Autodesk Inventor part; units mm, degrees
(part 2 of 2)
  line L549 (-543.4229, 5.588) -> (-545.3351, 0.3343)
  arc A272 (-545.8125, 0) -> (-545.3351, 0.3343) centre (-545.8125, 0.508) ccw
  line L550 (-545.8125, 0) -> (-547.3989, 0)
  arc A273 (-547.8763, 0.3343) -> (-547.3989, 0) centre (-547.3989, 0.508) ccw
  line L551 (-547.8763, 0.3343) -> (-549.7885, 5.588)
  arc A274 (-539.8966, 0.3343) -> (-539.4193, 0) centre (-539.4193, 0.508) ccw
  line L552 (-537.8328, 0) -> (-539.4193, 0)
  arc A275 (-537.8328, 0) -> (-537.3555, 0.3343) centre (-537.8328, 0.508) ccw
  line L553 (-535.4433, 5.588) -> (-537.3555, 0.3343)
  line L554 (-543.4229, 5.588) -> (-541.8088, 5.588)
  line L555 (-547.8763, 0.3343) -> (-549.7885, 5.588)
  line L556 (-554.5854, 0) -> (-546.6057, 0) construction
  line L557 (-551.4026, 5.588) -> (-553.3148, 0.3343)
  arc A276 (-553.7921, 0) -> (-553.3148, 0.3343) centre (-553.7921, 0.508) ccw
  line L558 (-553.7921, 0) -> (-555.3786, 0)
  arc A277 (-555.8559, 0.3343) -> (-555.3786, 0) centre (-555.3786, 0.508) ccw
  line L559 (-555.8559, 0.3343) -> (-557.7681, 5.588)
  arc A278 (-547.8763, 0.3343) -> (-547.3989, 0) centre (-547.3989, 0.508) ccw
  line L560 (-545.8125, 0) -> (-547.3989, 0)
  arc A279 (-545.8125, 0) -> (-545.3351, 0.3343) centre (-545.8125, 0.508) ccw
  line L561 (-543.4229, 5.588) -> (-545.3351, 0.3343)
  line L562 (-551.4026, 5.588) -> (-549.7885, 5.588)
  line L563 (7.1726, 38.1) -> (7.1726, 44.1)
  line L564 (7.1726, 44.1) -> (19.8726, 44.1)
  line L565 (19.8726, 44.1) -> (19.8726, -6)
  line L566 (19.8726, -6) -> (7.1726, -6)
  line L567 (7.1726, -6) -> (7.1726, 0)
  line L568 (4.783, 0) -> (7.1726, 0)
  point P0 (0, 0)
  point P1 (0, 0)
  point P2 (0, 5.588)
  point P3 (0, 0)
  point P4 (-7.9796, 5.588)
  point P5 (-7.9796, 0)
  point P6 (-7.9796, 0)
  point P7 (-7.9796, 0)
  point P8 (-15.9593, 5.588)
  point P9 (-15.9593, 0)
  point P10 (-15.9593, 0)
  point P11 (-15.9593, 0)
  point P12 (-23.9389, 5.588)
  point P13 (-23.9389, 0)
  point P14 (-23.9389, 0)
  point P15 (-23.9389, 0)
  point P16 (-31.9186, 5.588)
  point P17 (-31.9186, 0)
  point P18 (-31.9186, 0)
  point P19 (-31.9186, 0)
  point P20 (-39.8982, 5.588)
  point P21 (-39.8982, 0)
  point P22 (-39.8982, 0)
  point P23 (-39.8982, 0)
  point P24 (-47.8779, 5.588)
  point P25 (-47.8779, 0)
  point P26 (-47.8779, 0)
  point P27 (-47.8779, 0)
  point P28 (-55.8575, 5.588)
  point P29 (-55.8575, 0)
  point P30 (-55.8575, 0)
  point P31 (-55.8575, 0)
  point P32 (-63.8372, 5.588)
  point P33 (-63.8372, 0)
  point P34 (-63.8372, 0)
  point P35 (-63.8372, 0)
  point P36 (-71.8168, 5.588)
  point P37 (-71.8168, 0)
  point P38 (-71.8168, 0)
  point P39 (-71.8168, 0)
  point P40 (-79.7965, 5.588)
  point P41 (-79.7965, 0)
  point P42 (-79.7965, 0)
  point P43 (-79.7965, 0)
  point P44 (-87.7761, 5.588)
  point P45 (-87.7761, 0)
  point P46 (-87.7761, 0)
  point P47 (-87.7761, 0)
  point P48 (-95.7557, 5.588)
  point P49 (-95.7557, 0)
  point P50 (-95.7557, 0)
  point P51 (-95.7557, 0)
  point P52 (-103.7354, 5.588)
  point P53 (-103.7354, 0)
  point P54 (-103.7354, 0)
  point P55 (-103.7354, 0)
  point P56 (-111.715, 5.588)
  point P57 (-111.715, 0)
  point P58 (-111.715, 0)
  point P59 (-111.715, 0)
  point P60 (-119.6947, 5.588)
  point P61 (-119.6947, 0)
  point P62 (-119.6947, 0)
  point P63 (-119.6947, 0)
  point P64 (-127.6743, 5.588)
  point P65 (-127.6743, 0)
  point P66 (-127.6743, 0)
  point P67 (-127.6743, 0)
  point P68 (-135.654, 5.588)
  point P69 (-135.654, 0)
  point P70 (-135.654, 0)
  point P71 (-135.654, 0)
  point P72 (-143.6336, 5.588)
  point P73 (-143.6336, 0)
  point P74 (-143.6336, 0)
  point P75 (-143.6336, 0)
  point P76 (-151.6133, 5.588)
  point P77 (-151.6133, 0)
  point P78 (-151.6133, 0)
  point P79 (-151.6133, 0)
  point P80 (-159.5929, 5.588)
  point P81 (-159.5929, 0)
  point P82 (-159.5929, 0)
  point P83 (-159.5929, 0)
  point P84 (-167.5726, 5.588)
  point P85 (-167.5726, 0)
  point P86 (-167.5726, 0)
  point P87 (-167.5726, 0)
  point P88 (-175.5522, 5.588)
  point P89 (-175.5522, 0)
  point P90 (-175.5522, 0)
  point P91 (-175.5522, 0)
  point P92 (-183.5318, 5.588)
  point P93 (-183.5318, 0)
  point P94 (-183.5318, 0)
  point P95 (-183.5318, 0)
  point P96 (-191.5115, 5.588)
  point P97 (-191.5115, 0)
  point P98 (-191.5115, 0)
  point P99 (-191.5115, 0)
  point P100 (-199.4911, 5.588)
  point P101 (-199.4911, 0)
  point P102 (-199.4911, 0)
  point P103 (-199.4911, 0)
  point P104 (-207.4708, 5.588)
  point P105 (-207.4708, 0)
  point P106 (-207.4708, 0)
  point P107 (-207.4708, 0)
  point P108 (-215.4504, 5.588)
  point P109 (-215.4504, 0)
  point P110 (-215.4504, 0)
  point P111 (-215.4504, 0)
  point P112 (-223.4301, 5.588)
  point P113 (-223.4301, 0)
  point P114 (-223.4301, 0)
  point P115 (-223.4301, 0)
  point P116 (-231.4097, 5.588)
  point P117 (-231.4097, 0)
  point P118 (-231.4097, 0)
  point P119 (-231.4097, 0)
  point P120 (-239.3894, 5.588)
  point P121 (-239.3894, 0)
  point P122 (-239.3894, 0)
  point P123 (-239.3894, 0)
  point P124 (-247.369, 5.588)
  point P125 (-247.369, 0)
  point P126 (-247.369, 0)
  point P127 (-247.369, 0)
  point P128 (-255.3487, 5.588)
  point P129 (-255.3487, 0)
  point P130 (-255.3487, 0)
  point P131 (-255.3487, 0)
  point P132 (-263.3283, 5.588)
  point P133 (-263.3283, 0)
  point P134 (-263.3283, 0)
  point P135 (-263.3283, 0)
  point P136 (-271.3079, 5.588)
  point P137 (-271.3079, 0)
  point P138 (-271.3079, 0)
  point P139 (-271.3079, 0)
  point P140 (-279.2876, 5.588)
  point P141 (-279.2876, 0)
  point P142 (-279.2876, 0)
  point P143 (-279.2876, 0)
  point P144 (-287.2672, 5.588)
  point P145 (-287.2672, 0)
  point P146 (-287.2672, 0)
  point P147 (-287.2672, 0)
  point P148 (-295.2469, 5.588)
  point P149 (-295.2469, 0)
  point P150 (-295.2469, 0)
  point P151 (-295.2469, 0)
  point P152 (-303.2265, 5.588)
  point P153 (-303.2265, 0)
  point P154 (-303.2265, 0)
  point P155 (-303.2265, 0)
  point P156 (-311.2062, 5.588)
  point P157 (-311.2062, 0)
  point P158 (-311.2062, 0)
  point P159 (-311.2062, 0)
  point P160 (-319.1858, 5.588)
  point P161 (-319.1858, 0)
  point P162 (-319.1858, 0)
  point P163 (-319.1858, 0)
  point P164 (-327.1655, 5.588)
  point P165 (-327.1655, 0)
  point P166 (-327.1655, 0)
  point P167 (-327.1655, 0)
  point P168 (-335.1451, 5.588)
  point P169 (-335.1451, 0)
  point P170 (-335.1451, 0)
  point P171 (-335.1451, 0)
  point P172 (-343.1247, 5.588)
  point P173 (-343.1247, 0)
  point P174 (-343.1247, 0)
  point P175 (-343.1247, 0)
  point P176 (-351.1044, 5.588)
  point P177 (-351.1044, 0)
  point P178 (-351.1044, 0)
  point P179 (-351.1044, 0)
  point P180 (-359.084, 5.588)
  point P181 (-359.084, 0)
  point P182 (-359.084, 0)
  point P183 (-359.084, 0)
  point P184 (-367.0637, 5.588)
  point P185 (-367.0637, 0)
  point P186 (-367.0637, 0)
  point P187 (-367.0637, 0)
  point P188 (-375.0433, 5.588)
  point P189 (-375.0433, 0)
  point P190 (-375.0433, 0)
  point P191 (-375.0433, 0)
  point P192 (-383.023, 5.588)
  point P193 (-383.023, 0)
  point P194 (-383.023, 0)
  point P195 (-383.023, 0)
  point P196 (-391.0026, 5.588)
  point P197 (-391.0026, 0)
  point P198 (-391.0026, 0)
  point P199 (-391.0026, 0)
  dimension "d15" = 40
  dimension "d16" = 40
  dimension "d17" = 40
  dimension "d18" = 5.588
  dimension "d19" = 0.508
  dimension "d20" = 7.9796
  dimension "d21" = 3.9898
  dimension "d22" = 1.6141
  dimension "d23" = 1.5864
  dimension "d27" = 7.9796
  dimension "d32" = 38.1
  dimension "d35" = 6
  dimension "d36" = 6
  dimension "d37" = 12.7
  constraints: 1138 end point, 560 point on circle, 280 centre point, 141 coincident, 8 tangent, 7 perpendicular, 4 horizontal alignment, 4 midpoint, 3 equal radius, 2 horizontal, 2 point on line, 2 vertical, 1 collinear, 1 vertical alignment, 2346 other
  measures "d15" angle of L4 L6
  measures "d16" angle of L2 L4
  measures "d17" angle of L0 L2
  measures "d18" distance between parallel lines of L1 L3
  measures "d19" radius of A3
  measures "d20" distance of L7.end L7.start
  measures "d21" horizontal distance of point (0, 5.588) L7.start
  measures "d22" distance of L4.start L2.end
  measures "d23" distance of A2.centre A3.centre
  measures "d27" distance of L2.end L11.end
  measures "d32" distance between parallel lines of L444 L9
  measures "d35" distance of L8.end L563.end
  measures "d36" distance from line of L1.start L566
  measures "d37" distance of L563.end L564.end
extrude "Extrusion1" add sketch "Sketch1" along normal blind 4.7625
sketch "Sketch2" plane through (0, 0, 4.7625) normal (0, 0, 1) x (1, 0, 0)
  line L0 (7.1726, 2.54) -> (-557.7681, 2.54) construction
  line L1 (-555.3786, 0) -> (-553.7921, 0) projected
  point P0 (0, 0)
  point P1 (-557.7681, 5.588)
  point P2 (-554.5854, 0)
  point P3 (7.1726, 0)
  dimension "d39" = 2.54
  constraints: 2 end point, 2 vertical alignment, 1 horizontal, 1 midpoint
  measures "d39" distance from line of point (-554.585, 0) L0
fillet "Fillet1" radius 3 6 edges at (7.1726, 38.1, 2.3813) (7.1726, 44.1, 2.3813) (19.8726, 44.1, 2.3813) (19.8726, -6, 2.3813) (7.1726, -6, 2.3813) (7.1726, 0, 2.3813)
body "Solid1"
